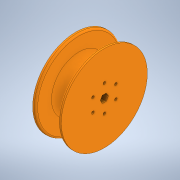
# Autodesk Inventor part: WheelForHangingAndMoving
Saved by Autodesk Inventor 2020.2 (Build 242310000, 310)
## iProperties
Created: 2020-01-06
Part Number: WheelForHangingAndMoving
Material: PBT Plastic
Document SubType Name: Modeling
Designer: steele
Density: 1.31 g/cm^3
Appearance: Orange
Author: steele
Autodesk Inventor part; units mm, degrees
ref_plane "YZ Plane" through (0, 0, 0) normal (1, 0, 0) x (0, 1, 0)
ref_plane "XZ Plane" through (0, 0, 0) normal (0, 1, 0) x (-1, 0, 0)
ref_plane "XY Plane" through (0, 0, 0) normal (0, 0, 1) x (1, 0, 0)
sketch "Sketch1" plane through (0, 0, 0) normal (0, 0, 1) x (1, 0, 0)
  arc A0 (-21.082, 52.832) -> (21.082, 52.832) centre (0, 52.832) ccw
  line L0 (-21.082, 52.832) -> (-21.082, 0)
  line L1 (21.082, 52.832) -> (21.082, 0)
  line L2 (-21.082, 0) -> (21.082, 0)
  line L3 (-21.082, 0) -> (-27.432, 0)
  line L4 (-27.432, 0) -> (-27.432, 82.55)
  line L5 (-27.432, 82.55) -> (-24.257, 82.55)
  line L6 (-21.082, 79.375) -> (-21.082, 0)
  line L7 (21.082, 0) -> (27.432, 0)
  line L8 (27.432, 0) -> (27.432, 82.55)
  line L9 (27.432, 82.55) -> (24.257, 82.55)
  line L10 (21.082, 79.375) -> (21.082, 0)
  line L11 (0, 0) -> (-27.432, 0) construction
  arc A1 (24.257, 82.55) -> (21.082, 79.375) centre (24.257, 79.375) ccw
  arc A2 (-21.082, 79.375) -> (-24.257, 82.55) centre (-24.257, 79.375) ccw
  point P0 (-21.082, 82.55)
  point P1 (21.082, 82.55)
  dimension "diameterOfPipe" = 42.164
  dimension "d6" = 6.35
  dimension "d8" = 6.35
  dimension "d27" = 82.55
  dimension "d28" = 52.832
  dimension "d29" = 31.75
  dimension "d30" = 3.175
  constraints: 24 end point, 6 point on circle, 5 point on line, 5 tangent, 4 parallel, 3 centre point, 3 horizontal, 3 perpendicular, 2 collinear, 2 vertical, 1 equal radius
  measures "diameterOfPipe" diameter of A0
  measures "d6" distance of L4.end point (-21.082, 82.55)
  measures "d8" distance of point (21.082, 82.55) L8.end
  measures "d27" distance between parallel lines of L9 L7
  measures "d28" distance of A0.centre L11.start
  measures "d29" distance edge to line of A0 L2
  measures "d30" radius of A1
revolve "Revolution1" add sketch "Sketch1" angle 360 about axis through (-21.082, 0, 0) along (1, 0, 0)
sketch "Sketch3" plane through (27.432, 0, 0) normal (1, 0, 0) x (0, 0, -1)
  line L0 (7.9189, 0) -> (3.9595, -6.858)
  line L1 (3.9595, -6.858) -> (-3.9595, -6.858)
  line L2 (-3.9595, -6.858) -> (-7.9189, 0)
  line L3 (-7.9189, 0) -> (-3.9595, 6.858)
  line L4 (-3.9595, 6.858) -> (3.9595, 6.858)
  line L5 (3.9595, 6.858) -> (7.9189, 0)
  point P0 (0, 0)
  point P1 (0, 0)
  dimension "hexWidth" = 13.716
  constraints: 12 end point, 1 coincident, 1 horizontal, 13 other
  measures "hexWidth" distance between parallel lines of L1 L4
extrude "Extrusion2" cut sketch "Sketch3" against normal through all
sketch "Sketch4" plane through (27.432, 0, 0) normal (1, 0, 0) x (0, 0, -1)
  point P0 (0, 0)
  point P1 (0, 25.4)
  point P2 (-21.997, 12.7)
  point P3 (-21.997, -12.7)
  point P4 (0, -25.4)
  point P5 (21.997, -12.7)
  point P6 (21.997, 12.7)
  dimension "d14" = 25.4
  dimension "d17" = 360
  constraints: 7 other
  measures "d14" distance of point (0, 25.4) point (0, 0)
hole "Hole1" at (27.432, 25.4, 0) at (27.432, 12.7, 21.997) at (27.432, -12.7, 21.997) at (27.432, -25.4, 0) at (27.432, -12.7, -21.997) at (27.432, 12.7, -21.997) direction (-1, 0, 0) diameter 5.1054 end through all clearance for "Flat Head Machine Screw (82)" size "#10" standard "Ansi Unified Screw Threads"
equation "\"d6\" = widthOfOutside"
equation "\"d8\" = widthOfOutside"
equation "\"widthOfOutside\" = 6.35"
body "Solid1"
